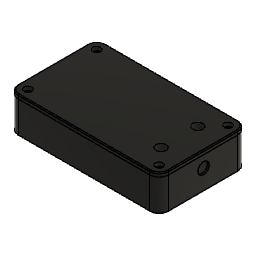
8.4V_Charger_Case (Autodesk Fusion 360 design; units mm, degrees)
Autodesk Fusion 360 part; units mm, degrees
sketch "Sketch1" plane through (0, 0, 0) normal (0, 0, 1) x (1, 0, 0)
  line L0 (37.7, -21.2) -> (-37.7, -21.2)
  line L1 (-37.7, -21.2) -> (-37.7, 21.2)
  line L2 (-37.7, 21.2) -> (37.7, 21.2)
  line L3 (37.7, 21.2) -> (37.7, -21.2)
  line L4 (37.7, -21.2) -> (-37.7, 21.2) construction
  line L5 (-37.7, -21.2) -> (37.7, 21.2) construction
  line L6 (39.7, -23.2) -> (-39.7, -23.2)
  line L7 (-39.7, -23.2) -> (-39.7, 23.2)
  line L8 (-39.7, 23.2) -> (39.7, 23.2)
  line L9 (39.7, 23.2) -> (39.7, -23.2)
  line L10 (39.7, -23.2) -> (-39.7, 23.2) construction
  line L11 (-39.7, -23.2) -> (39.7, 23.2) construction
  dimension "d1" = 75.4
  dimension "d2" = 42.4
  dimension "d3" = 79.4
  dimension "d4" = 46.4
  constraint horizontal L0
  constraint perpendicular L0 L1
  constraint parallel L0 L2
  constraint parallel L1 L3
  constraint coincident L4 origin
  constraint coincident L5 origin
  constraint horizontal L6
  constraint perpendicular L6 L7
  constraint parallel L6 L8
  constraint parallel L7 L9
  constraint coincident L10 origin
  constraint coincident L11 origin
  measures "d1" distance of L1.end L2.end
  measures "d2" distance of L0.end L1.end
  measures "d3" distance of L7.end L8.end
  measures "d4" distance of L6.end L7.end
extrude "Extrude1" add sketch "Sketch1" along normal blind 2 contours L0 L1 L2 L3 makes body 1
extrude "Extrude2" add sketch "Sketch1" along normal blind 17 bodies 1
sketch "Sketch2" plane through (0, 0, 2) normal (0, 0, 1) x (-1, 0, 0)
  line L0 (-37.7, -21.2) -> (37.7, -21.2)
  line L1 (37.7, -21.2) -> (37.7, 21.2)
  line L2 (37.7, 21.2) -> (-37.7, 21.2)
  line L3 (-37.7, 21.2) -> (-37.7, -21.2)
  line L4 (37.5, -21) -> (-37.5, -21)
  line L5 (-37.5, -21) -> (-37.5, 21)
  line L6 (-37.5, 21) -> (37.5, 21)
  line L7 (37.5, 21) -> (37.5, -21)
  line L8 (37.5, -21) -> (-37.5, 21) construction
  line L9 (-37.5, -21) -> (37.5, 21) construction
  line L10 (-1.0419, 21) -> (-1.0419, -21)
  dimension "d9" = 75
  dimension "d10" = 42
  constraint horizontal L4
  constraint perpendicular L4 L5
  constraint parallel L4 L6
  constraint parallel L5 L7
  constraint coincident L8 origin
  constraint coincident L9 origin
  constraint coincident L6 L10.start
  constraint coincident L4 L10.end
  constraint perpendicular L4 L10
  measures "d9" distance of L5.end L6.end
  measures "d10" distance of L4.end L5.end
sketch "Sketch3" plane through (37.7, 0, 0) normal (-1, 0, 0) x (0, -1, 0)
  line L0 (-21.2, 2) -> (21.2, 2)
  line L1 (21.2, 2) -> (21.2, 17)
  line L2 (21.2, 17) -> (-21.2, 17)
  line L3 (-21.2, 17) -> (-21.2, 2)
  circle A0 centre (-0.2425, 10.8598) radius 3
  line L4 (-4.3225, 15.3398) -> (3.8375, 15.3398)
  line L5 (-4.6225, 4.7398) -> (-4.6225, 15.0398)
  line L6 (4.1375, 15.0398) -> (4.1375, 4.7398)
  line L7 (3.8375, 4.5398) -> (-4.3225, 4.5398)
  line L8 (4.1375, 15.0398) -> (4.1375, 15.3398)
  line L9 (4.1375, 15.3398) -> (3.8375, 15.3398)
  line L10 (-4.3225, 15.3398) -> (-4.6225, 15.3398)
  line L11 (-4.6225, 15.3398) -> (-4.6225, 15.0398)
  line L12 (-4.6225, 4.7398) -> (-4.6225, 4.5398)
  line L13 (-4.6225, 4.5398) -> (-4.3225, 4.5398)
  line L14 (4.1375, 4.7398) -> (4.1375, 4.5398)
  line L15 (4.1375, 4.5398) -> (3.8375, 4.5398)
  line L16 (3.8375, 4.3398) -> (-4.3225, 4.3398)
  line L17 (-4.8225, 4.3398) -> (-4.3225, 4.3398)
  line L18 (-4.8225, 4.7398) -> (-4.8225, 4.3398)
  line L19 (-4.8225, 4.7398) -> (-4.8225, 15.0398)
  line L20 (-4.8225, 15.5398) -> (-4.8225, 15.0398)
  line L21 (-4.3225, 15.5398) -> (-4.8225, 15.5398)
  line L22 (-4.3225, 15.5398) -> (3.8375, 15.5398)
  line L23 (4.3375, 15.5398) -> (3.8375, 15.5398)
  line L24 (4.3375, 15.0398) -> (4.3375, 15.5398)
  line L25 (4.3375, 15.0398) -> (4.3375, 4.7398)
  line L26 (4.3375, 4.7398) -> (4.3375, 4.3398)
  line L27 (4.3375, 4.3398) -> (3.8375, 4.3398)
  dimension "d11" = -0.2
  constraint coincident L6.start L8.start
  constraint perpendicular L4 L8
  constraint coincident L4.end L9.end
  constraint perpendicular L6 L9
  constraint coincident L4.start L10.start
  constraint perpendicular L5 L10
  constraint coincident L5.end L11.end
  constraint perpendicular L10 L11
  constraint coincident L5.start L12.start
  constraint perpendicular L7 L12
  constraint coincident L7.end L13.end
  constraint perpendicular L12 L13
  constraint coincident L6.end L14.start
  constraint perpendicular L7 L14
  constraint coincident L7.start L15.end
  constraint perpendicular L14 L15
extrude "Extrude3" cut sketch "Sketch3" against normal blind 2 contours A0 bodies 1
extrude "Extrude4" cut sketch "Sketch3" against normal blind 1 contours L4 L5 L6 L7 L8 L9 L10 L11 L12 L13 L14 L15 | L16 L17 L18 L19 L20 L21 L22 L23 L24 L25 L26 L27 bodies 1
sketch "Sketch4" plane through (-39.7, 0, 0) normal (-1, 0, 0) x (0, -1, 0)
  line L0 (-23.2, 0) -> (23.2, 0)
  line L1 (23.2, 0) -> (23.2, 17)
  line L2 (23.2, 17) -> (-23.2, 17)
  line L3 (-23.2, 17) -> (-23.2, 0)
  circle A0 centre (0, 10) radius 1.75
  point P0 (0, 10)
  dimension "d16" = 3.5
  dimension "d36" = 10
  constraint coincident P0 A0.centre
  measures "d16" diameter of A0
  measures "d36" distance of L0 P0
extrude "Extrude5" cut sketch "Sketch4" against normal blind 2 contours A0 bodies 1
sketch "Sketch5" plane through (-37.7, 0, 0) normal (1, 0, 0) x (0, 1, 0)
  circle A0 centre (0, 10) radius 1.75
  line L0 (-21.2, 2) -> (21.2, 2)
  line L1 (21.2, 2) -> (21.2, 17)
  line L2 (21.2, 17) -> (-21.2, 17)
  line L3 (-21.2, 17) -> (-21.2, 2)
  line L4 (-21.2, 17) -> (-13.7, 17)
  line L5 (-13.7, 17) -> (-13.7, 15)
  line L6 (-13.7, 15) -> (-21.2, 15)
  line L7 (-21.2, 15) -> (-21.2, 17)
  dimension "d19" = 7.5
  dimension "d20" = 2
  constraint horizontal L4
  constraint vertical L5
  constraint horizontal L6
  constraint vertical L7
  constraint coincident L2.end L3.start
  measures "d19" distance of L2.end L4.end
  measures "d20" distance of L2.end L6.end
extrude "Extrude6" add sketch "Sketch5" along normal blind 7.5 contours L2 L3 L4 L5 L6 L7 bodies 1
fillet "Fillet1" radius 3.75 1 edges at (-30.2, -13.7, 16) on bodies 1
sketch "Sketch6" plane through (0, 0, 17) normal (0, 0, 1) x (-1, 0, 0)
  line L0 (-39.7, -23.2) -> (39.7, -23.2)
  line L1 (39.7, -23.2) -> (39.7, 23.2)
  line L2 (39.7, 23.2) -> (-39.7, 23.2)
  line L3 (-39.7, 23.2) -> (-39.7, -23.2)
  arc A0 (30.2, 17.45) -> (33.95, 13.7) centre (33.95, 17.45) ccw
  line L4 (33.95, 13.7) -> (37.7, 13.7)
  line L5 (37.7, 13.7) -> (37.7, -21.2)
  line L6 (37.7, -21.2) -> (-37.7, -21.2)
  line L7 (-37.7, -21.2) -> (-37.7, 21.2)
  line L8 (-37.7, 21.2) -> (30.2, 21.2)
  line L9 (30.2, 21.2) -> (30.2, 17.45)
  circle A1 centre (34.7, 18.2) radius 1.25
  dimension "d25" = 2.5
  dimension "d26" = 5
  dimension "d27" = 5
  measures "d25" diameter of A1
  measures "d26" distance of L1 A1.centre
  measures "d27" distance of L2 A1.centre
sketch "Sketch10" plane through (-37.7, 0, 0) normal (1, 0, 0) x (0, 1, 0)
  line L0 (-13.7, 17) -> (-13.7, 15)
  line L1 (-13.7, 15) -> (-21.2, 15)
  line L2 (-21.2, 15) -> (-21.2, 2)
  line L3 (-21.2, 2) -> (21.2, 2)
  line L4 (21.2, 2) -> (21.2, 17)
  line L5 (21.2, 17) -> (-13.7, 17)
  circle A0 centre (0, 10) radius 1.75
  point P0 (-21.2, 10.4428)
  constraint coincident L2 P0
loft "Loft1" add section 1 point at (-37.7, -21.2, 10.4428) section 2 face at (-33.95, -17.45, 15) on bodies 1 bodies 1
extrude "Extrude7" cut sketch "Sketch6" against normal blind 6 contours A1 bodies 1
mirror "Mirror1" about plane through (0, 0, 0) normal (0, 1, 0) of "Extrude6", "Fillet1", "Loft1", "Extrude7"
mirror "Mirror2" about plane through (0, 0, 0) normal (1, 0, 0) of "Extrude6", "Fillet1", "Loft1", "Extrude7", "Mirror1"
sketch "Sketch7" plane through (0, 0, 17) normal (0, 0, 1) x (-1, 0, 0)
  circle A0 centre (-34.7, -18.2) radius 1.25
  line L0 (-39.7, -23.2) -> (39.7, -23.2)
  line L1 (39.7, -23.2) -> (39.7, 23.2)
  line L2 (39.7, 23.2) -> (-39.7, 23.2)
  line L3 (-39.7, 23.2) -> (-39.7, -23.2)
  circle A1 centre (34.7, 18.2) radius 1.25
  circle A2 centre (34.7, -18.2) radius 1.25
  arc A3 (-30.2, -17.45) -> (-33.95, -13.7) centre (-33.95, -17.45) ccw
  line L4 (-33.95, -13.7) -> (-37.7, -13.7)
  line L5 (-37.7, -13.7) -> (-37.7, 13.7)
  line L6 (-37.7, 13.7) -> (-33.95, 13.7)
  arc A4 (-33.95, 13.7) -> (-30.2, 17.45) centre (-33.95, 17.45) ccw
  line L7 (-30.2, 17.45) -> (-30.2, 21.2)
  line L8 (-30.2, 21.2) -> (30.2, 21.2)
  line L9 (30.2, 21.2) -> (30.2, 17.45)
  arc A5 (30.2, 17.45) -> (33.95, 13.7) centre (33.95, 17.45) ccw
  line L10 (33.95, 13.7) -> (37.7, 13.7)
  line L11 (37.7, 13.7) -> (37.7, -13.7)
  line L12 (37.7, -13.7) -> (33.95, -13.7)
  arc A6 (33.95, -13.7) -> (30.2, -17.45) centre (33.95, -17.45) ccw
  line L13 (30.2, -17.45) -> (30.2, -21.2)
  line L14 (30.2, -21.2) -> (-30.2, -21.2)
  line L15 (-30.2, -21.2) -> (-30.2, -17.45)
  circle A7 centre (-34.7, 18.2) radius 1.25
  line L16 (-39.7, 23.2) -> (39.7, 23.2)
  line L17 (39.7, 23.2) -> (39.7, -23.2)
  line L18 (39.7, -23.2) -> (-39.7, -23.2)
  line L19 (-39.7, -23.2) -> (-39.7, 23.2)
  constraint horizontal L16
  constraint vertical L17
  constraint horizontal L18
  constraint vertical L19
  constraint coincident L0.end L1.start
  constraint coincident L2.end L3.start
extrude "Extrude8" add sketch "Sketch7" along normal blind 2 separate body contours A0 | L0 L1 L2 L3 L16 L17 L18 L19 | A1 | A2 | A3 L4 L5 L6 A4 L7 L8 L9 A5 L10 L11 L12 A6 L13 L14 L15 | A7 makes body 2
sketch "Sketch8" plane through (0, 0, 19) normal (0, 0, 1) x (-1, 0, 0)
  line L0 (-39.7, -23.2) -> (39.7, -23.2)
  line L1 (39.7, -23.2) -> (39.7, 23.2)
  line L2 (39.7, 23.2) -> (-39.7, 23.2)
  line L3 (-39.7, 23.2) -> (-39.7, -23.2)
  circle A0 centre (-34.7, 18.2) radius 1.25
  circle A1 centre (-34.7, 18.2) radius 2
  dimension "d37" = 0.75
extrude "Extrude9" cut sketch "Sketch8" against normal blind 2 contours A0 | A1 bodies 2
mirror "Mirror3" about plane through (0, 0, 0) normal (0, 1, 0) of "Extrude9"
mirror "Mirror4" about plane through (0, 0, 0) normal (1, 0, 0) of "Extrude9", "Mirror3"
fillet "Fillet2" radius 5 8 edges at (-39.7, 23.2, 8.5) (-39.7, -23.2, 8.5) (39.7, 23.2, 8.5) (39.7, -23.2, 8.5) (-39.7, 23.2, 18) (-39.7, -23.2, 18) (39.7, 23.2, 18) (39.7, -23.2, 18) on bodies 1 2
sketch "Sketch9" plane through (0, 0, 17) normal (0, 0, -1) x (1, 0, 0)
  circle A0 centre (-34.7, -18.2) radius 2
  circle A1 centre (-34.7, 18.2) radius 2
  circle A2 centre (34.7, -18.2) radius 2
  circle A3 centre (34.7, 18.2) radius 2
  arc A4 (39.7, 18.2) -> (34.7, 23.2) centre (34.7, 18.2) ccw
  line L0 (34.7, 23.2) -> (-34.7, 23.2)
  arc A5 (-34.7, 23.2) -> (-39.7, 18.2) centre (-34.7, 18.2) ccw
  line L1 (-39.7, 18.2) -> (-39.7, -18.2)
  arc A6 (-39.7, -18.2) -> (-34.7, -23.2) centre (-34.7, -18.2) ccw
  line L2 (-34.7, -23.2) -> (34.7, -23.2)
  arc A7 (34.7, -23.2) -> (39.7, -18.2) centre (34.7, -18.2) ccw
  line L3 (39.7, -18.2) -> (39.7, 18.2)
  circle A8 centre (27.2, -9.7) radius 2.65
  circle A9 centre (27.2, -9.7) radius 3.45
  dimension "d46" = 5.3
  dimension "d48" = 13.5
  dimension "d49" = 0.8
  dimension "d64" = 12.5
  measures "d46" diameter of A8
  measures "d48" distance of L2 A8.centre
  measures "d64" distance of L3 A8.centre
extrude "Extrude10" cut sketch "Sketch9" against normal blind 2 contours A8 bodies 2
extrude "Extrude11" add sketch "Sketch9" along normal blind 5.8 contours A9 bodies 2
mirror "Mirror5" about plane through (0, 0, 0) normal (0, 1, 0) of "Extrude10", "Extrude11"
fillet "Fillet3" radius 0.5 16 edges at (38.2355, 21.7355, 0) (39.7, 0, 0) (38.2355, -21.7355, 0) (0, -23.2, 0) (-38.2355, -21.7355, 0) (-39.7, 0, 0) (-38.2355, 21.7355, 0) (0, 23.2, 0) (-38.2355, 21.7355, 19) (-39.7, 0, 19) (-38.2355, -21.7355, 19) (0, -23.2, 19) (38.2355, -21.7355, 19) (39.7, 0, 19) (38.2355, 21.7355, 19) (0, 23.2, 19) on bodies 1 2
fillet "Fillet4" radius 1 4 edges at (37.7, -21.2, 6.2214) (37.7, 21.2, 6.2214) (-37.7, 21.2, 6.2214) (-37.7, -21.2, 6.2214) on bodies 1
named bodies: "Case", "Cap"
